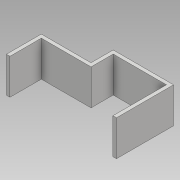
# Autodesk Inventor part: センサ冶具
Saved by Autodesk Inventor 2017 (Build 210142000, 142)
## iProperties
Part Number: センサ冶具
Material: 一般
Document SubType Name: Modeling
Designer: HISAAKI
Density: 1 g/cm^3
Appearance: 既定
Author: HISAAKI
Autodesk Inventor part; units mm, degrees
ref_plane "YZ Plane" through (0, 0, 0) normal (1, 0, 0) x (0, 1, 0)
ref_plane "XZ Plane" through (0, 0, 0) normal (0, 1, 0) x (-1, 0, 0)
ref_plane "XY Plane" through (0, 0, 0) normal (0, 0, 1) x (1, 0, 0)
sketch "スケッチ1" plane through (0, 0, 0) normal (0, 0, 1) x (1, 0, 0)
  line L0 (0, 0) -> (0, 17.65)
  line L1 (0, 17.65) -> (28, 17.65)
  line L2 (28, 17.65) -> (28, 30.15)
  line L3 (28, 30.15) -> (58, 30.15)
  line L4 (58, 30.15) -> (58, 0)
  line L5 (58, 0) -> (60, 0)
  line L6 (60, 0) -> (60, 32.15)
  line L7 (60, 32.15) -> (28, 32.15)
  line L8 (28, 32.15) -> (26, 32.15)
  line L9 (26, 32.15) -> (26, 19.65)
  line L10 (26, 19.65) -> (-2, 19.65)
  line L11 (-2, 19.65) -> (-2, 0)
  line L12 (-2, 0) -> (0, 0)
  dimension "d0" = 17.65
  dimension "d1" = 28
  dimension "d2" = 12.5
  dimension "d3" = 30
  dimension "d4" = 2
  dimension "d5" = 32.15
  dimension "d6" = 32
  dimension "d7" = 2
  dimension "d8" = 12.5
  dimension "d9" = 28
  constraints: 26 end point, 7 perpendicular, 3 parallel, 3 point on line, 1 vertical
  measures "d0" distance of L0.start L0.end
  measures "d1" distance of L0.end L1.end
  measures "d2" distance of L1.end L2.end
  measures "d3" distance of L2.end L3.end
  measures "d4" distance of L4.end L5.end
  measures "d5" distance of L5.end L6.end
  measures "d6" distance of L6.end L7.end
  measures "d7" distance of L7.end L8.end
  measures "d8" distance of L8.end L9.end
  measures "d9" distance of L9.end L10.end
extrude "押し出し1" add sketch "スケッチ1" along normal blind 20
